# Autodesk Inventor part: BRM-2A18VERT
Saved by Autodesk Inventor 2016 SP1 (Build 200210100, 210)
## iProperties
Created: 2015-11-19
Part Number: BRM-2A18VERT
Material: Generic
Document SubType Name: Modeling
Designer: PhillipD
Density: 1 g/cm^3
Appearance: BRM-2508_VERT, BRM-2A18VERT
Author: PhillipD
Autodesk Inventor part; units mm, degrees
ref_plane "YZ Plane" through (0, 0, 0) normal (1, 0, 0) x (0, 1, 0)
ref_plane "XZ Plane" through (0, 0, 0) normal (0, 1, 0) x (-1, 0, 0)
ref_plane "XY Plane" through (0, 0, 0) normal (0, 0, 1) x (1, 0, 0)
sketch "BRM-2508_VERT, BRM-2A18VERT_76" plane through (0, 0, 0) normal (0, 0, 1) x (1, 0, 0)
  line L0 (-3.69, 8.2435) -> (3.0635, 8.2435)
  line L1 (3.0635, 8.2435) -> (3.0635, -1.1)
  line L2 (3.0635, -1.1) -> (-3.69, -1.1)
  line L3 (-3.69, -1.1) -> (-3.69, 8.2435)
  constraints: 8 end point
extrude "Extrusion1" add sketch "BRM-2508_VERT, BRM-2A18VERT_76" along normal blind 1
body "Solid1"
